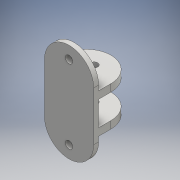
# Autodesk Inventor part: turretSupport
Saved by Autodesk Inventor 2016 (Build 200138000, 138)
## iProperties
Created: 2016-04-17
Part Number: turretSupport
Material: PC/ABS Plastic
Document SubType Name: Modeling
Designer: amenoni
Density: 0.357273 g/cm^3
Appearance: Smooth - White
Author: amenoni
Autodesk Inventor part; units mm, degrees
ref_plane "YZ Plane" through (0, 0, 0) normal (1, 0, 0) x (0, 1, 0)
ref_plane "XZ Plane" through (0, 0, 0) normal (0, 1, 0) x (-1, 0, 0)
ref_plane "XY Plane" through (0, 0, 0) normal (0, 0, 1) x (1, 0, 0)
sketch "Sketch1" plane through (0, 0, 0) normal (0, 1, 0) x (-1, 0, 0)
  line L0 (-10, -20) -> (10, -20)
  line L1 (10, -20) -> (10, 20)
  line L2 (10, 20) -> (-10, 20)
  line L3 (-10, 20) -> (-10, -20)
  line L4 (-10, -20) -> (10, 20) construction
  line L5 (10, -20) -> (-10, 20) construction
  point P0 (0, 0)
  dimension "d0" = 20
  dimension "d1" = 40
  constraints: 12 end point, 2 midpoint, 2 parallel, 1 horizontal, 1 perpendicular
  measures "d0" distance of L2.end L1.end
  measures "d1" distance of L1.end L0.end
extrude "Extrusion1" add sketch "Sketch1" along normal blind 2
sketch "Sketch3" plane through (0, 2, 0) normal (0, 1, 0) x (1, 0, 0)
  line L0 (-10, 20) -> (-10, -20) projected
  line L1 (10, -20) -> (10, 20) projected
  line L2 (-10, -8) -> (10, -8)
  line L3 (10, -8) -> (10, -5)
  line L4 (10, -5) -> (-10, -5)
  line L5 (-10, -5) -> (-10, -8)
  line L6 (-6.0097, 0) -> (5.0263, 0)
  line L7 (-10, 8) -> (10, 8)
  line L8 (10, 8) -> (10, 5)
  line L9 (10, 5) -> (-10, 5)
  line L10 (-10, 5) -> (-10, 8)
  point P0 (0, 0)
  dimension "d6" = 3
  dimension "d7" = 5
  constraints: 18 end point, 4 symmetric about line, 2 horizontal, 2 parallel, 2 point on line, 1 perpendicular
  measures "d6" distance of L3.end L2.end
  measures "d7" distance from line of point (0, 0) L4
extrude "Extrusion2" add sketch "Sketch3" along normal blind 15 contours L7 L1 L9 L0 | L4 L1 L2 L0
fillet "Fillet1" radius 10 4 edges at (10, 17, 6.5) (-10, 17, 6.5) (10, 17, -6.5) (-10, 17, -6.5)
sketch "Sketch4" plane through (0, 2, 0) normal (0, 1, 0) x (1, 0, 0)
  line L0 (10, 20) -> (-10, 20) projected
  line L1 (-10, -20) -> (10, -20) projected
  point P0 (0, 0)
  point P1 (0, 15)
  point P2 (0, -15)
  dimension "d11" = 5
  dimension "d12" = 5
  measures "d11" distance from line of point (0, 15) L0
  measures "d12" distance from line of L1 point (0, -15)
hole "Hole1" at (0, 2, -15) at (0, 2, 15) direction (0, -1, 0) diameter 3 end through all
fillet "Fillet2" radius 10 4 edges at (10, 1, 20) (-10, 1, 20) (-10, 1, -20) (10, 1, -20)
sketch "Sketch5" plane through (10, 2, -8) normal (0, 0, -1) x (-1, 0, 0)
  point P0 (10, -2)
  point P1 (10, 8.1411)
hole "Hole2" at (0, 10.1411, -8) direction (0, 0, 1) diameter 3 end through all
body "Solid1"
